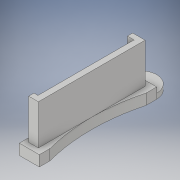
# Autodesk Inventor part: sem2_plateclip
Saved by Autodesk Inventor 2018 (Build 220112000, 112)
## iProperties
Created: 2018-03-15
Part Number: sem2_plateclip
Material: Generic
Document SubType Name: Modeling
Designer: rheal
Density: 1 g/cm^3
Appearance: Default
Author: rheal
Autodesk Inventor part; units mm, degrees
ref_plane "YZ Plane" through (0, 0, 0) normal (1, 0, 0) x (0, 1, 0)
ref_plane "XZ Plane" through (0, 0, 0) normal (0, 1, 0) x (-1, 0, 0)
ref_plane "XY Plane" through (0, 0, 0) normal (0, 0, 1) x (1, 0, 0)
sketch "Sketch1" plane through (0, 0, 0) normal (0, 1, 0) x (-1, 0, 0)
  line L0 (0, 0) -> (0, -36)
  line L1 (0, -36) -> (5, -36)
  line L2 (7.5, -40) -> (-4.5, -40)
  line L3 (-4.5, -40) -> (-4.5, -36)
  arc A0 (-4.5, -36) -> (-4.5, 0) centre (-72.1461, -18) ccw
  line L4 (-4.5, 0) -> (-4.5, 4)
  line L5 (-4.5, 4) -> (3, 4)
  line L6 (3, 4) -> (3, 0)
  line L7 (3, 0) -> (0, 0)
  line L8 (7.5, -40) -> (7.5, -10)
  line L9 (7.5, -10) -> (5, -10)
  line L10 (5, -10) -> (5, -36)
  dimension "d0" = 36
  dimension "d1" = 5
  dimension "d4" = 12
  dimension "d6" = 70
  dimension "d7" = 4
  dimension "d8" = 7.5
  dimension "d20" = 30
  constraints: 22 end point, 6 perpendicular, 4 vertical, 2 point on circle, 1 centre point, 1 point on line
  measures "d0" distance of L0.start L0.end
  measures "d1" distance of L0.end L1.end
  measures "d4" distance of L2.start L2.end
  measures "d6" radius of A0
  measures "d7" distance of L4.start L4.end
  measures "d8" distance of L4.end L5.end
  measures "d20" distance of L2.start L8.end
extrude "Extrusion1" add sketch "Sketch1" along normal blind 4
sketch "Sketch2" plane through (0, 0, 0) normal (0, -1, 0) x (1, 0, 0)
  line L0 (-7.5, -40) -> (4.5, -40) projected
  arc A0 (-7.5, -40) -> (4.5, -40) centre (-1.5, -40) ccw
  line L1 (4.5, -40) -> (-7.5, -40)
  point P0 (0, 0)
  constraints: 2 end point, 2 point on circle, 1 centre point, 1 collinear, 1 midpoint
extrude "Extrusion2" add sketch "Sketch2" against normal blind 2
sketch "Sketch3" plane through (0, 4, 0) normal (0, 1, 0) x (1, 0, 0)
  line L0 (0, 0) -> (-1.5, 0)
  line L1 (-3, 0) -> (0, 0) projected
  line L2 (-1.5, 0) -> (-1.5, -2)
  arc A0 (4.5, 36) -> (4.5, 0) centre (72.1461, 18) ccw projected
  line L3 (2.1461, 18) -> (2.1461, -2)
  line L4 (2.1461, -2) -> (-1.5, -2)
  line L5 (0, 36) -> (-5, 36) projected
  line L6 (-2.5, 36) -> (-2.5, 38)
  line L7 (2.1461, 18) -> (2.1461, 38)
  line L8 (2.1461, 38) -> (-2.5, 38)
  line L9 (0, 36) -> (0, 0) projected
  line L10 (0, 0) -> (0, 36)
  line L11 (0, 36) -> (-2.5, 36)
  dimension "d15" = 2
  dimension "d17" = 2
  constraints: 18 end point, 4 perpendicular, 3 vertical, 2 midpoint, 2 tangent, 1 collinear, 1 point on circle
  measures "d15" distance of L0.end L2.end
  measures "d17" distance of L6.start L6.end
extrude "Extrusion3" add sketch "Sketch3" along normal blind 15
body "Solid1"
